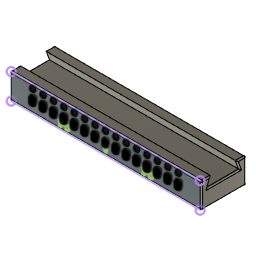
Sliding Mount (Autodesk Fusion 360 design; units mm, degrees)
Autodesk Fusion 360 part; units mm, degrees
sketch "Sketch1" plane through (0, 0, 0) normal (1, 0, 0) x (0, 1, 0)
  line L0 (0, 0) -> (35, 0)
  line L1 (35, 0) -> (35, 20)
  line L2 (35, 20) -> (0, 20)
  line L3 (0, 20) -> (0, 0)
  dimension "d1" = 35
  dimension "d2" = 20
  constraint horizontal L0
  constraint vertical L1
  constraint horizontal L2
  constraint vertical L3
  constraint coincident L0.start L3.end
  measures "d1" distance of L0.start L0.end
  measures "d2" distance of L0.start L2.end
extrude "Extrude1" add sketch "Sketch1" along normal blind 150
sketch "Mounting Point" plane through (0, 0, 0) normal (0, 0, -1) x (1, 0, 0)
  line L0 (0, 0) -> (0, -35)
  line L1 (0, -35) -> (150, -35)
  line L2 (150, -35) -> (150, 0)
  line L3 (150, 0) -> (0, 0)
  line L4 (63, -5.5) -> (87, -5.5)
  line L5 (87, -5.5) -> (87, -29.5)
  line L6 (87, -29.5) -> (63, -29.5)
  line L7 (63, -29.5) -> (63, -5.5)
  dimension "d17" = 24
  dimension "d18" = 24
  dimension "d19" = 5.5
  dimension "d20" = 63
  constraint horizontal L4
  constraint vertical L5
  constraint horizontal L6
  constraint vertical L7
  measures "d17" distance of L4.start L4.end
  measures "d18" distance of L4.start L6.end
  measures "d19" distance of L3 L4
  measures "d20" distance of L0 L7
sketch "Dovetail" plane through (150, 0, 0) normal (1, 0, 0) x (0, 1, 0)
  line L0 (0, 20) -> (0, 0)
  line L1 (0, 0) -> (35, 0)
  line L2 (35, 0) -> (35, 20)
  line L3 (35, 20) -> (0, 20)
  line L4 (7.5478, 20) -> (27.4522, 20)
  line L5 (30, 13) -> (5, 13)
  line L6 (5, 13) -> (7.5478, 20)
  line L7 (5, 13) -> (11.5169, 13) construction
  line L8 (30, 13) -> (27.4522, 20)
  line L9 (30, 13) -> (35.383, 13) construction
  dimension "d10" = 70
  dimension "d11" = 110
  dimension "d12" = 7
  dimension "d13" = 25
  dimension "d14" = 5
  constraint horizontal L4
  constraint horizontal L5
  constraint horizontal L7
  constraint horizontal L9
  measures "d10" angle of L6 L7
  measures "d11" angle of L8 L9
  measures "d12" distance of L4 L5
  measures "d13" distance of L5.start L5.end
  measures "d14" distance of L2 L5.start
extrude "Extrude2" cut sketch "Dovetail" against normal blind 151 contours L3 L4 L5 L6 L8
extrude "Extrude3" cut sketch "Mounting Point" against normal blind 10 contours L4 L5 L6 L7
fillet "Fillet1" radius 1 1 faces at (150, 13.3333, 4.3333)
fillet "Fillet2" radius 1 1 faces at (0, 13.3333, 4.3333)
fillet "Fillet3" radius 1 3 edges at (0.2929, 0.2929, 0.2929) (75, 0, 0) (149.7071, 0.2929, 0.2929)
fillet "Fillet4" radius 1 3 edges at (0.2929, 34.7071, 0.2929) (75, 35, 0) (149.7071, 34.7071, 0.2929)
fillet "Fillet5" radius 1 6 edges at (0.2929, 34.7071, 19.7071) (75, 35, 20) (149.7071, 34.7071, 19.7071) (0.2929, 0.2929, 19.7071) (75, 0, 20) (149.7071, 0.2929, 19.7071)
sketch "Sketch4" plane through (0, 0, 0) normal (0, -1, 0) x (1, 0, 0)
  line L0 (149, 19) -> (1, 19)
  line L1 (1, 19) -> (1, 1)
  line L2 (1, 1) -> (149, 1)
  line L3 (149, 1) -> (149, 19)
  line L4 (75.25, 10.5) -> (74.75, 10.5)
  line L5 (74.5, 10.25) -> (74.5, 7.75)
  line L6 (74.75, 7.5) -> (75.25, 7.5)
  line L7 (75.5, 7.75) -> (75.5, 10.25)
  line L8 (75.5, 10.5) -> (74.5, 7.5) construction
  line L9 (74.5, 10.5) -> (75.5, 7.5) construction
  arc A0 (74.75, 10.5) -> (74.5, 10.25) centre (74.75, 10.25) ccw
  arc A1 (74.5, 7.75) -> (74.75, 7.5) centre (74.75, 7.75) ccw
  arc A2 (75.25, 7.5) -> (75.5, 7.75) centre (75.25, 7.75) ccw
  arc A3 (75.5, 10.25) -> (75.25, 10.5) centre (75.25, 10.25) ccw
  line L10 (83.6429, 7.75) -> (83.6429, 10.25)
  arc A4 (83.3929, 7.5) -> (83.6429, 7.75) centre (83.3929, 7.75) ccw
  arc A5 (83.6429, 10.25) -> (83.3929, 10.5) centre (83.3929, 10.25) ccw
  line L11 (82.6429, 10.5) -> (83.6429, 7.5) construction
  line L12 (82.6429, 10.25) -> (82.6429, 7.75)
  arc A6 (82.6429, 7.75) -> (82.8929, 7.5) centre (82.8929, 7.75) ccw
  line L13 (82.8929, 7.5) -> (83.3929, 7.5)
  line L14 (83.6429, 10.5) -> (82.6429, 7.5) construction
  line L15 (83.3929, 10.5) -> (82.8929, 10.5)
  arc A7 (82.8929, 10.5) -> (82.6429, 10.25) centre (82.8929, 10.25) ccw
  line L16 (91.7857, 7.75) -> (91.7857, 10.25)
  arc A8 (91.5357, 7.5) -> (91.7857, 7.75) centre (91.5357, 7.75) ccw
  arc A9 (91.7857, 10.25) -> (91.5357, 10.5) centre (91.5357, 10.25) ccw
  line L17 (90.7857, 10.5) -> (91.7857, 7.5) construction
  line L18 (90.7857, 10.25) -> (90.7857, 7.75)
  arc A10 (90.7857, 7.75) -> (91.0357, 7.5) centre (91.0357, 7.75) ccw
  line L19 (91.0357, 7.5) -> (91.5357, 7.5)
  line L20 (91.7857, 10.5) -> (90.7857, 7.5) construction
  line L21 (91.5357, 10.5) -> (91.0357, 10.5)
  arc A11 (91.0357, 10.5) -> (90.7857, 10.25) centre (91.0357, 10.25) ccw
  line L22 (99.9286, 7.75) -> (99.9286, 10.25)
  arc A12 (99.6786, 7.5) -> (99.9286, 7.75) centre (99.6786, 7.75) ccw
  arc A13 (99.9286, 10.25) -> (99.6786, 10.5) centre (99.6786, 10.25) ccw
  line L23 (98.9286, 10.5) -> (99.9286, 7.5) construction
  line L24 (98.9286, 10.25) -> (98.9286, 7.75)
  arc A14 (98.9286, 7.75) -> (99.1786, 7.5) centre (99.1786, 7.75) ccw
  line L25 (99.1786, 7.5) -> (99.6786, 7.5)
  line L26 (99.9286, 10.5) -> (98.9286, 7.5) construction
  line L27 (99.6786, 10.5) -> (99.1786, 10.5)
  arc A15 (99.1786, 10.5) -> (98.9286, 10.25) centre (99.1786, 10.25) ccw
  line L28 (108.0714, 7.75) -> (108.0714, 10.25)
  arc A16 (107.8214, 7.5) -> (108.0714, 7.75) centre (107.8214, 7.75) ccw
  arc A17 (108.0714, 10.25) -> (107.8214, 10.5) centre (107.8214, 10.25) ccw
  line L29 (107.0714, 10.5) -> (108.0714, 7.5) construction
  line L30 (107.0714, 10.25) -> (107.0714, 7.75)
  arc A18 (107.0714, 7.75) -> (107.3214, 7.5) centre (107.3214, 7.75) ccw
  line L31 (107.3214, 7.5) -> (107.8214, 7.5)
  line L32 (108.0714, 10.5) -> (107.0714, 7.5) construction
  line L33 (107.8214, 10.5) -> (107.3214, 10.5)
  arc A19 (107.3214, 10.5) -> (107.0714, 10.25) centre (107.3214, 10.25) ccw
  line L34 (116.2143, 7.75) -> (116.2143, 10.25)
  arc A20 (115.9643, 7.5) -> (116.2143, 7.75) centre (115.9643, 7.75) ccw
  arc A21 (116.2143, 10.25) -> (115.9643, 10.5) centre (115.9643, 10.25) ccw
  line L35 (115.2143, 10.5) -> (116.2143, 7.5) construction
  line L36 (115.2143, 10.25) -> (115.2143, 7.75)
  arc A22 (115.2143, 7.75) -> (115.4643, 7.5) centre (115.4643, 7.75) ccw
  line L37 (115.4643, 7.5) -> (115.9643, 7.5)
  line L38 (116.2143, 10.5) -> (115.2143, 7.5) construction
  line L39 (115.9643, 10.5) -> (115.4643, 10.5)
  arc A23 (115.4643, 10.5) -> (115.2143, 10.25) centre (115.4643, 10.25) ccw
  line L40 (124.3571, 7.75) -> (124.3571, 10.25)
  arc A24 (124.1071, 7.5) -> (124.3571, 7.75) centre (124.1071, 7.75) ccw
  arc A25 (124.3571, 10.25) -> (124.1071, 10.5) centre (124.1071, 10.25) ccw
  line L41 (123.3571, 10.5) -> (124.3571, 7.5) construction
  line L42 (123.3571, 10.25) -> (123.3571, 7.75)
  arc A26 (123.3571, 7.75) -> (123.6071, 7.5) centre (123.6071, 7.75) ccw
  line L43 (123.6071, 7.5) -> (124.1071, 7.5)
  line L44 (124.3571, 10.5) -> (123.3571, 7.5) construction
  line L45 (124.1071, 10.5) -> (123.6071, 10.5)
  arc A27 (123.6071, 10.5) -> (123.3571, 10.25) centre (123.6071, 10.25) ccw
  line L46 (132.5, 7.75) -> (132.5, 10.25)
  arc A28 (132.25, 7.5) -> (132.5, 7.75) centre (132.25, 7.75) ccw
  arc A29 (132.5, 10.25) -> (132.25, 10.5) centre (132.25, 10.25) ccw
  line L47 (131.5, 10.5) -> (132.5, 7.5) construction
  line L48 (131.5, 10.25) -> (131.5, 7.75)
  arc A30 (131.5, 7.75) -> (131.75, 7.5) centre (131.75, 7.75) ccw
  line L49 (131.75, 7.5) -> (132.25, 7.5)
  line L50 (132.5, 10.5) -> (131.5, 7.5) construction
  line L51 (132.25, 10.5) -> (131.75, 10.5)
  arc A31 (131.75, 10.5) -> (131.5, 10.25) centre (131.75, 10.25) ccw
  line L52 (66.3571, 10.5) -> (67.3571, 7.5) construction
  line L53 (67.3571, 7.75) -> (67.3571, 10.25)
  arc A32 (67.3571, 10.25) -> (67.1071, 10.5) centre (67.1071, 10.25) ccw
  arc A33 (66.6071, 10.5) -> (66.3571, 10.25) centre (66.6071, 10.25) ccw
  arc A34 (67.1071, 7.5) -> (67.3571, 7.75) centre (67.1071, 7.75) ccw
  line L54 (66.6071, 7.5) -> (67.1071, 7.5)
  arc A35 (66.3571, 7.75) -> (66.6071, 7.5) centre (66.6071, 7.75) ccw
  line L55 (67.3571, 10.5) -> (66.3571, 7.5) construction
  line L56 (67.1071, 10.5) -> (66.6071, 10.5)
  line L57 (66.3571, 10.25) -> (66.3571, 7.75)
  line L58 (58.2143, 10.5) -> (59.2143, 7.5) construction
  line L59 (59.2143, 7.75) -> (59.2143, 10.25)
  arc A36 (59.2143, 10.25) -> (58.9643, 10.5) centre (58.9643, 10.25) ccw
  arc A37 (58.4643, 10.5) -> (58.2143, 10.25) centre (58.4643, 10.25) ccw
  arc A38 (58.9643, 7.5) -> (59.2143, 7.75) centre (58.9643, 7.75) ccw
  line L60 (58.4643, 7.5) -> (58.9643, 7.5)
  arc A39 (58.2143, 7.75) -> (58.4643, 7.5) centre (58.4643, 7.75) ccw
  line L61 (59.2143, 10.5) -> (58.2143, 7.5) construction
  line L62 (58.9643, 10.5) -> (58.4643, 10.5)
  line L63 (58.2143, 10.25) -> (58.2143, 7.75)
  line L64 (50.0714, 10.5) -> (51.0714, 7.5) construction
  line L65 (51.0714, 7.75) -> (51.0714, 10.25)
  arc A40 (51.0714, 10.25) -> (50.8214, 10.5) centre (50.8214, 10.25) ccw
  arc A41 (50.3214, 10.5) -> (50.0714, 10.25) centre (50.3214, 10.25) ccw
  arc A42 (50.8214, 7.5) -> (51.0714, 7.75) centre (50.8214, 7.75) ccw
  line L66 (50.3214, 7.5) -> (50.8214, 7.5)
  arc A43 (50.0714, 7.75) -> (50.3214, 7.5) centre (50.3214, 7.75) ccw
  line L67 (51.0714, 10.5) -> (50.0714, 7.5) construction
  line L68 (50.8214, 10.5) -> (50.3214, 10.5)
  line L69 (50.0714, 10.25) -> (50.0714, 7.75)
  line L70 (41.9286, 10.5) -> (42.9286, 7.5) construction
  line L71 (42.9286, 7.75) -> (42.9286, 10.25)
  arc A44 (42.9286, 10.25) -> (42.6786, 10.5) centre (42.6786, 10.25) ccw
  arc A45 (42.1786, 10.5) -> (41.9286, 10.25) centre (42.1786, 10.25) ccw
  arc A46 (42.6786, 7.5) -> (42.9286, 7.75) centre (42.6786, 7.75) ccw
  line L72 (42.1786, 7.5) -> (42.6786, 7.5)
  arc A47 (41.9286, 7.75) -> (42.1786, 7.5) centre (42.1786, 7.75) ccw
  line L73 (42.9286, 10.5) -> (41.9286, 7.5) construction
  line L74 (42.6786, 10.5) -> (42.1786, 10.5)
  line L75 (41.9286, 10.25) -> (41.9286, 7.75)
  line L76 (33.7857, 10.5) -> (34.7857, 7.5) construction
  line L77 (34.7857, 7.75) -> (34.7857, 10.25)
  arc A48 (34.7857, 10.25) -> (34.5357, 10.5) centre (34.5357, 10.25) ccw
  arc A49 (34.0357, 10.5) -> (33.7857, 10.25) centre (34.0357, 10.25) ccw
  arc A50 (34.5357, 7.5) -> (34.7857, 7.75) centre (34.5357, 7.75) ccw
  line L78 (34.0357, 7.5) -> (34.5357, 7.5)
  arc A51 (33.7857, 7.75) -> (34.0357, 7.5) centre (34.0357, 7.75) ccw
  line L79 (34.7857, 10.5) -> (33.7857, 7.5) construction
  line L80 (34.5357, 10.5) -> (34.0357, 10.5)
  line L81 (33.7857, 10.25) -> (33.7857, 7.75)
  line L82 (25.6429, 10.5) -> (26.6429, 7.5) construction
  line L83 (26.6429, 7.75) -> (26.6429, 10.25)
  arc A52 (26.6429, 10.25) -> (26.3929, 10.5) centre (26.3929, 10.25) ccw
  arc A53 (25.8929, 10.5) -> (25.6429, 10.25) centre (25.8929, 10.25) ccw
  arc A54 (26.3929, 7.5) -> (26.6429, 7.75) centre (26.3929, 7.75) ccw
  line L84 (25.8929, 7.5) -> (26.3929, 7.5)
  arc A55 (25.6429, 7.75) -> (25.8929, 7.5) centre (25.8929, 7.75) ccw
  line L85 (26.6429, 10.5) -> (25.6429, 7.5) construction
  line L86 (26.3929, 10.5) -> (25.8929, 10.5)
  line L87 (25.6429, 10.25) -> (25.6429, 7.75)
  line L88 (17.5, 10.5) -> (18.5, 7.5) construction
  line L89 (18.5, 7.75) -> (18.5, 10.25)
  arc A56 (18.5, 10.25) -> (18.25, 10.5) centre (18.25, 10.25) ccw
  arc A57 (17.75, 10.5) -> (17.5, 10.25) centre (17.75, 10.25) ccw
  arc A58 (18.25, 7.5) -> (18.5, 7.75) centre (18.25, 7.75) ccw
  line L90 (17.75, 7.5) -> (18.25, 7.5)
  arc A59 (17.5, 7.75) -> (17.75, 7.5) centre (17.75, 7.75) ccw
  line L91 (18.5, 10.5) -> (17.5, 7.5) construction
  line L92 (18.25, 10.5) -> (17.75, 10.5)
  line L93 (17.5, 10.25) -> (17.5, 7.75)
  line L94 (1, 0) -> (149, 0)
  spline S0 degree 2 poles (73.678, 4.2855) (73.678, 4.9949) (73.824, 5.4274) knots 0 0 0 1 1 1
  spline S1 degree 2 poles (73.824, 5.4274) (73.97, 5.8598) (74.2578, 6.0945) knots 0 0 0 1 1 1
  spline S2 degree 2 poles (74.2578, 6.0945) (74.5457, 6.3291) (74.9823, 6.3291) knots 0 0 0 1 1 1
  spline S3 degree 2 poles (74.9823, 6.3291) (75.3042, 6.3291) (75.5471, 6.1995) knots 0 0 0 1 1 1
  spline S4 degree 2 poles (75.5471, 6.1995) (75.7899, 6.0699) (75.9482, 5.8257) knots 0 0 0 1 1 1
  spline S5 degree 2 poles (75.9482, 5.8257) (76.1064, 5.5815) (76.1965, 5.2309) knots 0 0 0 1 1 1
  spline S6 degree 2 poles (76.1965, 5.2309) (76.2865, 4.8803) (76.2865, 4.2855) knots 0 0 0 1 1 1
  spline S7 degree 2 poles (76.2865, 4.2855) (76.2865, 3.5815) (76.1419, 3.149) knots 0 0 0 1 1 1
  spline S8 degree 2 poles (76.1419, 3.149) (75.9973, 2.7166) (75.7094, 2.4806) knots 0 0 0 1 1 1
  spline S9 degree 2 poles (75.7094, 2.4806) (75.4216, 2.2445) (74.9823, 2.2445) knots 0 0 0 1 1 1
  spline S10 degree 2 poles (74.9823, 2.2445) (74.4038, 2.2445) (74.0737, 2.6593) knots 0 0 0 1 1 1
  spline S11 degree 2 poles (74.0737, 2.6593) (73.678, 3.1586) (73.678, 4.2855) knots 0 0 0 1 1 1
  spline S12 degree 2 poles (74.1828, 4.2855) (74.1828, 3.3005) (74.4134, 2.9744) knots 0 0 0 1 1 1
  spline S13 degree 2 poles (74.4134, 2.9744) (74.6439, 2.6484) (74.9823, 2.6484) knots 0 0 0 1 1 1
  spline S14 degree 2 poles (74.9823, 2.6484) (75.3206, 2.6484) (75.5512, 2.9758) knots 0 0 0 1 1 1
  spline S15 degree 2 poles (75.5512, 2.9758) (75.7817, 3.3032) (75.7817, 4.2855) knots 0 0 0 1 1 1
  spline S16 degree 2 poles (75.7817, 4.2855) (75.7817, 5.2732) (75.5512, 5.5979) knots 0 0 0 1 1 1
  spline S17 degree 2 poles (75.5512, 5.5979) (75.3206, 5.9226) (74.9768, 5.9226) knots 0 0 0 1 1 1
  spline S18 degree 2 poles (74.9768, 5.9226) (74.6385, 5.9226) (74.4366, 5.6361) knots 0 0 0 1 1 1
  spline S19 degree 2 poles (74.4366, 5.6361) (74.1828, 5.2705) (74.1828, 4.2855) knots 0 0 0 1 1 1
  line L95 (103.7744, 2.037) -> (103.7814, 6.037)
  line L96 (103.7814, 6.037) -> (104.3108, 6.0361)
  line L97 (104.3108, 6.0361) -> (104.3038, 2.0361)
  line L98 (104.3038, 2.0361) -> (103.7744, 2.037)
  line L99 (105.2369, 2.0344) -> (105.2439, 6.0344)
  line L100 (105.2439, 6.0344) -> (106.7528, 6.0318)
  spline S20 degree 2 poles (106.7528, 6.0318) (107.1512, 6.0311) (107.3612, 5.9925) knots 0 0 0 1 1 1
  spline S21 degree 2 poles (107.3612, 5.9925) (107.6558, 5.9429) (107.8547, 5.8048) knots 0 0 0 1 1 1
  spline S22 degree 2 poles (107.8547, 5.8048) (108.0537, 5.6666) (108.1746, 5.4181) knots 0 0 0 1 1 1
  spline S23 degree 2 poles (108.1746, 5.4181) (108.2956, 5.1696) (108.2951, 4.8722) knots 0 0 0 1 1 1
  spline S24 degree 2 poles (108.2951, 4.8722) (108.2942, 4.362) (107.9689, 4.0092) knots 0 0 0 1 1 1
  spline S25 degree 2 poles (107.9689, 4.0092) (107.6436, 3.6564) (106.795, 3.6579) knots 0 0 0 1 1 1
  line L101 (106.795, 3.6579) -> (105.7691, 3.6597)
  line L102 (105.7691, 3.6597) -> (105.7663, 2.0335)
  line L103 (105.7663, 2.0335) -> (105.2369, 2.0344)
  line L104 (105.7699, 4.1317) -> (106.804, 4.1299)
  spline S26 degree 2 poles (106.804, 4.1299) (107.317, 4.129) (107.5329, 4.3196) knots 0 0 0 1 1 1
  spline S27 degree 2 poles (107.5329, 4.3196) (107.7488, 4.5103) (107.7494, 4.8568) knots 0 0 0 1 1 1
  spline S28 degree 2 poles (107.7494, 4.8568) (107.7498, 5.1078) (107.6232, 5.2867) knots 0 0 0 1 1 1
  spline S29 degree 2 poles (107.6232, 5.2867) (107.4967, 5.4657) (107.2894, 5.5233) knots 0 0 0 1 1 1
  spline S30 degree 2 poles (107.2894, 5.5233) (107.1558, 5.559) (106.7956, 5.5597) knots 0 0 0 1 1 1
  line L105 (106.7956, 5.5597) -> (105.7724, 5.5615)
  line L106 (105.7724, 5.5615) -> (105.7699, 4.1317)
  line L107 (108.9641, 2.0279) -> (108.9711, 6.0279)
  line L108 (108.9711, 6.0279) -> (110.349, 6.0255)
  spline S31 degree 2 poles (110.349, 6.0255) (110.8155, 6.0247) (111.061, 5.9669) knots 0 0 0 1 1 1
  spline S32 degree 2 poles (111.061, 5.9669) (111.4047, 5.8872) (111.6471, 5.6794) knots 0 0 0 1 1 1
  spline S33 degree 2 poles (111.6471, 5.6794) (111.9632, 5.4115) (112.1193, 4.9951) knots 0 0 0 1 1 1
  spline S34 degree 2 poles (112.1193, 4.9951) (112.2755, 4.5787) (112.2746, 4.0439) knots 0 0 0 1 1 1
  spline S35 degree 2 poles (112.2746, 4.0439) (112.2738, 3.5883) (112.1667, 3.2365) knots 0 0 0 1 1 1
  spline S36 degree 2 poles (112.1667, 3.2365) (112.0597, 2.8847) (111.8929, 2.6544) knots 0 0 0 1 1 1
  spline S37 degree 2 poles (111.8929, 2.6544) (111.726, 2.4242) (111.528, 2.2922) knots 0 0 0 1 1 1
  spline S38 degree 2 poles (111.528, 2.2922) (111.3299, 2.1602) (111.0501, 2.0925) knots 0 0 0 1 1 1
  spline S39 degree 2 poles (111.0501, 2.0925) (110.7703, 2.0247) (110.4074, 2.0254) knots 0 0 0 1 1 1
  line L109 (110.4074, 2.0254) -> (108.9641, 2.0279)
  line L110 (109.4942, 2.499) -> (110.3482, 2.4975)
  spline S40 degree 2 poles (110.3482, 2.4975) (110.7439, 2.4968) (110.9691, 2.5701) knots 0 0 0 1 1 1
  spline S41 degree 2 poles (110.9691, 2.5701) (111.1943, 2.6434) (111.3283, 2.7768) knots 0 0 0 1 1 1
  spline S42 degree 2 poles (111.3283, 2.7768) (111.5169, 2.9648) (111.6225, 3.2825) knots 0 0 0 1 1 1
  spline S43 degree 2 poles (111.6225, 3.2825) (111.7281, 3.6001) (111.7289, 4.0531) knots 0 0 0 1 1 1
  spline S44 degree 2 poles (111.7289, 4.0531) (111.73, 4.6806) (111.5246, 5.018) knots 0 0 0 1 1 1
  spline S45 degree 2 poles (111.5246, 5.018) (111.3191, 5.3553) (111.0247, 5.4704) knots 0 0 0 1 1 1
  spline S46 degree 2 poles (111.0247, 5.4704) (110.812, 5.5526) (110.34, 5.5535) knots 0 0 0 1 1 1
  line L111 (110.34, 5.5535) -> (109.4996, 5.5549)
  line L112 (109.4996, 5.5549) -> (109.4942, 2.499)
  line L113 (38.321, 2) -> (38.321, 6)
  line L114 (38.321, 6) -> (38.8504, 6)
  line L115 (38.8504, 6) -> (38.8504, 2)
  line L116 (38.8504, 2) -> (38.321, 2)
  line L117 (39.7835, 2) -> (39.7835, 6)
  line L118 (39.7835, 6) -> (41.2924, 6)
  spline S47 degree 2 poles (41.2924, 6) (41.6908, 6) (41.9008, 5.9618) knots 0 0 0 1 1 1
  spline S48 degree 2 poles (41.9008, 5.9618) (42.1955, 5.9127) (42.3947, 5.7749) knots 0 0 0 1 1 1
  spline S49 degree 2 poles (42.3947, 5.7749) (42.5939, 5.6371) (42.7153, 5.3888) knots 0 0 0 1 1 1
  spline S50 degree 2 poles (42.7153, 5.3888) (42.8367, 5.1405) (42.8367, 4.8431) knots 0 0 0 1 1 1
  spline S51 degree 2 poles (42.8367, 4.8431) (42.8367, 4.3329) (42.512, 3.9795) knots 0 0 0 1 1 1
  spline S52 degree 2 poles (42.512, 3.9795) (42.1873, 3.6262) (41.3388, 3.6262) knots 0 0 0 1 1 1
  line L119 (41.3388, 3.6262) -> (40.3129, 3.6262)
  line L120 (40.3129, 3.6262) -> (40.3129, 2)
  line L121 (40.3129, 2) -> (39.7835, 2)
  line L122 (40.3129, 4.0982) -> (41.347, 4.0982)
  spline S53 degree 2 poles (41.347, 4.0982) (41.8599, 4.0982) (42.0755, 4.2892) knots 0 0 0 1 1 1
  spline S54 degree 2 poles (42.0755, 4.2892) (42.291, 4.4802) (42.291, 4.8267) knots 0 0 0 1 1 1
  spline S55 degree 2 poles (42.291, 4.8267) (42.291, 5.0778) (42.1641, 5.2565) knots 0 0 0 1 1 1
  spline S56 degree 2 poles (42.1641, 5.2565) (42.0373, 5.4352) (41.8299, 5.4925) knots 0 0 0 1 1 1
  spline S57 degree 2 poles (41.8299, 5.4925) (41.6962, 5.528) (41.336, 5.528) knots 0 0 0 1 1 1
  line L123 (41.336, 5.528) -> (40.3129, 5.528)
  line L124 (40.3129, 5.528) -> (40.3129, 4.0982)
  line L125 (43.5107, 2) -> (43.5107, 6)
  line L126 (43.5107, 6) -> (44.8886, 6)
  spline S58 degree 2 poles (44.8886, 6) (45.3551, 6) (45.6007, 5.9427) knots 0 0 0 1 1 1
  spline S59 degree 2 poles (45.6007, 5.9427) (45.9445, 5.8636) (46.1873, 5.6562) knots 0 0 0 1 1 1
  spline S60 degree 2 poles (46.1873, 5.6562) (46.5038, 5.3888) (46.6607, 4.9727) knots 0 0 0 1 1 1
  spline S61 degree 2 poles (46.6607, 4.9727) (46.8176, 4.5566) (46.8176, 4.0218) knots 0 0 0 1 1 1
  spline S62 degree 2 poles (46.8176, 4.0218) (46.8176, 3.5662) (46.7112, 3.2142) knots 0 0 0 1 1 1
  spline S63 degree 2 poles (46.7112, 3.2142) (46.6048, 2.8622) (46.4384, 2.6317) knots 0 0 0 1 1 1
  spline S64 degree 2 poles (46.4384, 2.6317) (46.2719, 2.4011) (46.0741, 2.2688) knots 0 0 0 1 1 1
  spline S65 degree 2 poles (46.0741, 2.2688) (45.8763, 2.1364) (45.5966, 2.0682) knots 0 0 0 1 1 1
  spline S66 degree 2 poles (45.5966, 2.0682) (45.3169, 2) (44.9541, 2) knots 0 0 0 1 1 1
  line L127 (44.9541, 2) -> (43.5107, 2)
  line L128 (44.04, 2.472) -> (44.894, 2.472)
  spline S67 degree 2 poles (44.894, 2.472) (45.2897, 2.472) (45.5148, 2.5457) knots 0 0 0 1 1 1
  spline S68 degree 2 poles (45.5148, 2.5457) (45.7399, 2.6194) (45.8736, 2.7531) knots 0 0 0 1 1 1
  spline S69 degree 2 poles (45.8736, 2.7531) (46.0618, 2.9413) (46.1669, 3.2592) knots 0 0 0 1 1 1
  spline S70 degree 2 poles (46.1669, 3.2592) (46.2719, 3.5771) (46.2719, 4.03) knots 0 0 0 1 1 1
  spline S71 degree 2 poles (46.2719, 4.03) (46.2719, 4.6576) (46.0659, 4.9945) knots 0 0 0 1 1 1
  spline S72 degree 2 poles (46.0659, 4.9945) (45.8599, 5.3315) (45.5652, 5.4461) knots 0 0 0 1 1 1
  spline S73 degree 2 poles (45.5652, 5.4461) (45.3524, 5.528) (44.8804, 5.528) knots 0 0 0 1 1 1
  line L129 (44.8804, 5.528) -> (44.04, 5.528)
  line L130 (44.04, 5.528) -> (44.04, 2.472)
  line L131 (149, 20) -> (1, 20)
  circle A60 centre (75, 16.85) radius 2
  circle A61 centre (83.1429, 16.85) radius 2
  circle A62 centre (91.2857, 16.85) radius 2
  circle A63 centre (99.4286, 16.85) radius 2
  circle A64 centre (107.5714, 16.85) radius 2
  circle A65 centre (115.7143, 16.85) radius 2
  circle A66 centre (123.8571, 16.85) radius 2
  circle A67 centre (132, 16.85) radius 2
  circle A68 centre (66.8571, 16.85) radius 2
  circle A69 centre (58.7143, 16.85) radius 2
  circle A70 centre (50.5714, 16.85) radius 2
  circle A71 centre (42.4286, 16.85) radius 2
  circle A72 centre (34.2857, 16.85) radius 2
  circle A73 centre (26.1429, 16.85) radius 2
  circle A74 centre (18, 16.85) radius 2
  point P0 (75, 9)
  point P1 (83.1429, 9)
  point P2 (91.2857, 9)
  point P3 (99.4286, 9)
  point P4 (107.5714, 9)
  point P5 (115.7143, 9)
  point P6 (123.8571, 9)
  point P7 (132, 9)
  point P8 (66.8571, 9)
  point P9 (58.7143, 9)
  point P10 (50.5714, 9)
  point P11 (42.4286, 9)
  point P12 (34.2857, 9)
  point P13 (26.1429, 9)
  point P14 (18, 9)
  dimension "d35" = 1
  dimension "d36" = 3
  dimension "d37" = 0.25
  dimension "d38" = 74
  dimension "d39" = 8
  dimension "d44" = 57
  dimension "d45" = 0
  dimension "d48" = -57
  dimension "d49" = 0
  dimension "d67" = 4
  dimension "d69" = 3.15
  dimension "d70" = 74
  dimension "d77" = 57
  dimension "d78" = 0
  dimension "d81" = -57
  dimension "d82" = 0
  constraint horizontal L4
  constraint perpendicular L4 L5
  constraint parallel L4 L6
  constraint parallel L5 L7
  constraint coincident L8 P0
  constraint coincident L9 P0
  constraint coincident L9.start L4
  constraint coincident L9.start L5
  constraint tangent L4 A0
  constraint tangent L5 A0
  constraint coincident L8.end L5
  constraint coincident L8.end L6
  constraint tangent L5 A1
  constraint tangent L6 A1
  constraint equal A0 A1
  constraint coincident L9.end L6
  constraint coincident L9.end L7
  constraint tangent L6 A2
  constraint tangent L7 A2
  constraint equal A0 A2
  constraint coincident L8.start L7
  constraint coincident L8.start L4
  constraint tangent L7 A3
  constraint tangent L4 A3
  constraint equal A0 A3
  measures "d35" distance of L8.end L9.end
  measures "d36" distance of L9.start L8.end
  measures "d37" radius of A0
  measures "d38" distance of L3 P0
  measures "d39" distance of L2 P0
  measures "d67" diameter of A60
  measures "d69" distance of L131 A60.centre
  measures "d70" distance of L3 A60.centre
